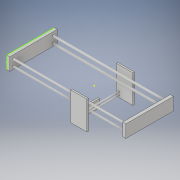
# Autodesk Inventor part: carving machine
Saved by Autodesk Inventor 2019 (Build 230136000, 136)
## iProperties
Created: 2019-10-09
Part Number: carving machine
Material: Generic
Document SubType Name: Modeling
Designer: Parasaram
Density: 1 g/cm^3
Appearance: Default
Author: Parasaram
Autodesk Inventor part; units mm, degrees
ref_plane "YZ Plane" through (0, 0, 0) normal (1, 0, 0) x (0, 1, 0)
ref_plane "XZ Plane" through (0, 0, 0) normal (0, 1, 0) x (-1, 0, 0)
ref_plane "XY Plane" through (0, 0, 0) normal (0, 0, 1) x (1, 0, 0)
sketch "Sketch1" plane through (0, 0, 0) normal (1, 0, 0) x (0, 1, 0)
  line L0 (4.0704, 14.9312) -> (-3.8604, 14.9312)
  line L1 (-3.8604, 14.9312) -> (-3.8604, -14.9567)
  line L2 (-3.8604, -14.9567) -> (4.0704, -14.9567)
  line L3 (4.0704, -14.9567) -> (4.0704, 14.9312)
  line L4 (4.0704, 14.9312) -> (-3.8604, -14.9567) construction
  line L5 (-3.8604, 14.9312) -> (4.0704, -14.9567) construction
  point P0 (0, 0)
  point P1 (0.105, -0.0127)
  constraints: 12 end point, 2 midpoint, 2 parallel, 1 horizontal, 1 perpendicular
extrude "Extrusion1" add sketch "Sketch1" along normal blind 2
sketch "Sketch2" plane through (2, 0, 0) normal (1, 0, 0) x (0, 0, -1)
  circle A0 centre (-12.7263, 1.8639) radius 0.5218
  circle A1 centre (-12.7263, -2.188) radius 0.5223
  circle A2 centre (12.3117, 1.8639) radius 0.5902
  circle A3 centre (12.3117, -2.188) radius 0.6302
  point P0 (0, 0)
  constraints: 4 centre point
extrude "Extrusion2" add sketch "Sketch2" along normal blind 71
sketch "Sketch3" plane through (73, 1.8639, 12.7263) normal (1, 0, 0) x (0, 0, -1)
  line L0 (-2.2049, 2.2065) -> (-2.2049, -5.7243) projected
  line L1 (-2.2049, -5.7243) -> (27.683, -5.7243) projected
  line L2 (-2.2049, 2.2065) -> (27.683, 2.2065)
  line L3 (27.683, 2.2065) -> (27.683, -5.7243)
  line L4 (27.683, -5.7243) -> (-2.2049, -5.7243)
  line L5 (-2.2049, -5.7243) -> (-2.2049, 2.2065)
  point P0 (12.7263, -1.8639)
  constraints: 8 end point, 2 parallel, 1 horizontal, 1 perpendicular
extrude "Extrusion3" add sketch "Sketch3" along normal blind 2
sketch "Sketch4" plane through (0, -3.8604, 14.9312) normal (0, 0, 1) x (1, 0, 0)
  point P0 (0, 3.8604)
sketch "Sketch5" plane through (73, -3.8604, 14.9312) normal (0, 0, 1) x (1, 0, 0)
  line L0 (-22.4506, -8.7315) -> (-32.8047, -8.7315)
  line L1 (-32.8047, -8.7315) -> (-32.8047, 9.0871)
  line L2 (-32.8047, 9.0871) -> (-22.4506, 9.0871)
  line L3 (-22.4506, 9.0871) -> (-22.4506, -8.7315)
  point P0 (-73, 3.8604)
  constraints: 8 end point, 2 parallel, 1 horizontal, 1 perpendicular
extrude "Extrusion4" add sketch "Sketch5" against normal blind 1
sketch "Sketch6" plane through (73, -3.8604, -14.9567) normal (0, 0, -1) x (-1, 0, 0)
  line L0 (22.4506, -8.7315) -> (32.8047, -8.7315) projected
  line L1 (32.8047, -8.7315) -> (22.4506, -8.7315)
  line L2 (22.4506, -8.7315) -> (22.4506, 9.0145)
  line L3 (22.4506, 9.0145) -> (32.8047, 9.0145)
  line L4 (32.8047, 9.0145) -> (32.8047, -8.7315)
  point P0 (73, 3.8604)
  constraints: 8 end point, 2 parallel, 1 horizontal, 1 perpendicular
extrude "Extrusion5" add sketch "Sketch6" against normal blind 1
sketch "Sketch7" plane through (73, -3.8604, 13.9312) normal (0, 0, -1) x (-1, 0, 0)
  circle A0 centre (31.234, -7.4132) radius 0.4052
  point P0 (73, 3.8604)
  constraints: 1 centre point
extrude "Extrusion6" add sketch "Sketch7" along normal blind 28
sketch "Sketch8" plane through (73, -3.8604, 13.9312) normal (0, 0, -1) x (-1, 0, 0)
  circle A0 centre (31.234, -5.6095) radius 0.4446
  point P0 (73, 3.8604)
  constraints: 1 centre point
extrude "Extrusion7" add sketch "Sketch8" along normal blind 28
sketch "Sketch9" plane through (40.1953, -12.5919, -14.9567) normal (-1, 0, 0) x (0, 0, 1)
  point P0 (14.9567, 12.5919)
sketch "Sketch10" plane through (40.1953, -12.5919, 14.9312) normal (-1, 0, 0) x (0, 0, 1)
  line L0 (-9.8431, 4.9293) -> (-17.303, 4.9293)
  line L1 (-17.303, 4.9293) -> (-17.303, -0.0575)
  line L2 (-17.303, -0.0575) -> (-9.8431, -0.0575)
  line L3 (-9.8431, -0.0575) -> (-9.8431, 4.9293)
  point P0 (-14.9312, 12.5919)
  constraints: 8 end point, 2 parallel, 1 horizontal, 1 perpendicular
extrude "Extrusion8" add sketch "Sketch10" against normal blind 1
body "Solid1"
